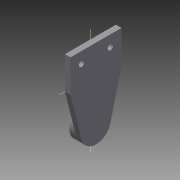
# Autodesk Inventor part: collar
Saved by Autodesk Inventor 2015 (Build 190159000, 159)
## iProperties
Created: 2015-09-23
Part Number: collar
Material: Generic
Description: insert part description/title
Document SubType Name: Modeling
Designer: francis
Density: 1 g/cm^3
Appearance: Default
Part Category: insert part category here and press enter to fill value
Author: francis
Autodesk Inventor part; units mm, degrees
ref_plane "YZ Plane" through (0, 0, 0) normal (1, 0, 0) x (0, 1, 0)
ref_plane "XZ Plane" through (0, 0, 0) normal (0, 1, 0) x (-1, 0, 0)
ref_plane "XY Plane" through (0, 0, 0) normal (0, 0, 1) x (1, 0, 0)
sketch "Sketch1" plane through (0, 0, 0) normal (1, 0, 0) x (0, 1, 0)
  line L0 (27.5, 35) -> (-27.5, 35)
  line L1 (-27.5, 35) -> (-27.5, 0)
  line L2 (-27.5, 0) -> (-15.5217, -47.8829)
  arc A0 (-15.5217, -47.8829) -> (15.5217, -47.8829) centre (0, -44) ccw
  line L3 (27.5, 35) -> (27.5, 0)
  line L4 (27.5, 0) -> (15.5217, -47.8829)
  line L5 (-38.5, 0) -> (38.5, 0) construction
  line L6 (0, -79) -> (0, 54) construction
  circle A1 centre (0, -44) radius 9
  point P0 (0, 0)
  point P1 (0, -60)
  dimension "d0" = 55
  dimension "d1" = 35
  dimension "d2" = 18
  dimension "d3" = 16
  dimension "d4" = 60
  constraints: 10 end point, 4 point on line, 3 point on circle, 2 centre point, 2 coincident, 2 tangent, 1 horizontal, 1 perpendicular, 1 vertical
  measures "d0" distance of L0.start L0.end
  measures "d1" distance of L0.end L1.end
  measures "d2" diameter of A1
  measures "d3" radius of A0
  measures "d4" distance from line of L5 point (0, -60)
extrude "Extrusion1" add sketch "Sketch1" along normal blind 6 contours L3 L4 A0 L2 L1 L0 | A1
sketch "Sketch2" plane through (0, 0, 0) normal (-1, 0, 0) x (0, 0, 1)
  circle A0 centre (-44.1499, 0) radius 15.8501
  arc A1 (-47.8829, 15.5217) -> (-47.8829, -15.5217) centre (-44, 0) ccw construction
  point P0 (0, 0)
  constraints: 1 centre point, 1 tangent
extrude "Extrusion2" add sketch "Sketch2" along normal blind 7
hole "Hole1" at (0, 15.5, 23) direction (1, 0, 0) diameter 6 end through all
hole "Hole2" at (0, -15.5, 23) direction (1, 0, 0) diameter 6 end through all
body "Solid1"
